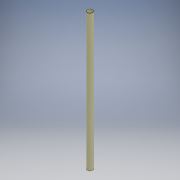
# Autodesk Inventor part: STK00-001
Saved by Autodesk Inventor 2018 (Build 220112000, 112)
## iProperties
Created: 2018-02-13
Part Number: STK00-001
Material: Polypropylene
Document SubType Name: Modeling
Designer: JARVIS
Mass: 214.535 g
Surface Area: 2390.89 cm^2
Volume: 238.637 cm^3
Density: 0.899 g/cm^3
Appearance: Smooth - Ash
Title: Body
Author: JARVIS
Autodesk Inventor part; units mm, degrees
ref_plane "YZ Plane" through (0, 0, 0) normal (1, 0, 0) x (0, 1, 0)
ref_plane "XZ Plane" through (0, 0, 0) normal (0, 1, 0) x (-1, 0, 0)
ref_plane "XY Plane" through (0, 0, 0) normal (0, 0, 1) x (1, 0, 0)
sketch "Sketch1" plane through (0, 0, 0) normal (0, 0, 1) x (1, 0, 0)
  circle A0 centre (0, 0) radius 20
  circle A1 centre (0, 0) radius 18
  dimension "d0" = 40
  dimension "d1" = 2
  constraints: 2 centre point, 1 coincident
  measures "d0" diameter of A0
  measures "d1" radial gap between concentric circles of A0 A1
extrude "Extrusion1" add sketch "Sketch1" along normal blind 1000
chamfer "Chamfer1" distance 1 angle 45 1 edges at (-20, 0, 1000)
chamfer "Chamfer2" distance 1 angle 45 1 edges at (-20, 0, 0)
body "Solid1"
